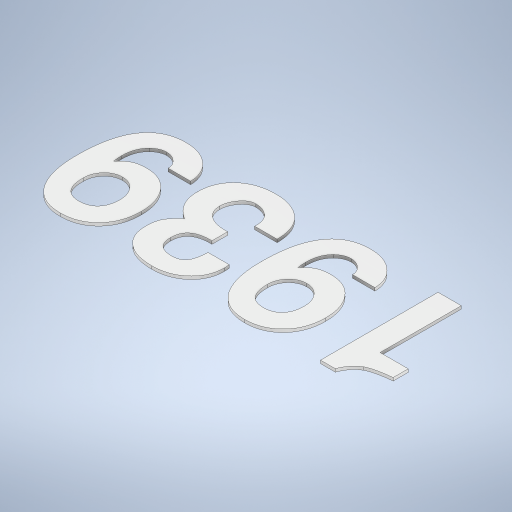
# Autodesk Inventor part: Numbers
Saved by Autodesk Inventor 2023 (Build 270158000, 158)
## iProperties
Created: 2023-11-22
Part Number: Numbers
Material: Generic
Document SubType Name: Modeling
Designer: adamarnold
Density: 1 g/cm^3
Appearance: Default
Author: adamarnold
Autodesk Inventor part; units mm, degrees
ref_plane "YZ Plane" through (0, 0, 0) normal (1, 0, 0) x (0, 1, 0)
ref_plane "XZ Plane" through (0, 0, 0) normal (0, 1, 0) x (-1, 0, 0)
ref_plane "XY Plane" through (0, 0, 0) normal (0, 0, 1) x (1, 0, 0)
sketch "Sketch1" plane through (0, 0, 0) normal (0, 1, 0) x (-1, 0, 0)
  line L0 (0, 0.0214) -> (189.558, 0.0214) construction
  line L1 (189.558, 0.0214) -> (189.558, -78.5059) construction
  line L2 (189.558, -78.5059) -> (0, -78.5059) construction
  line L3 (0, -78.5059) -> (0, 0.0214) construction
  line L4 (26.3876, -50.5021) -> (16.6305, -50.5021)
  line L5 (16.6305, -50.5021) -> (16.6305, -16.3721)
  line L6 (16.6305, -16.3721) -> (4.7798, -16.3721)
  line L7 (4.7798, -16.3721) -> (4.7798, -10.0122)
  spline S0 degree 2 poles (4.7798, -10.0122) (11.8112, -9.3012) (14.8134, -7.7606) knots 0 0 0 1 1 1
  spline S1 degree 2 poles (14.8134, -7.7606) (18.2896, -5.904) (20.1857, -1.0847) knots 0 0 0 1 1 1
  line L8 (20.1857, -1.0847) -> (26.3876, -1.0847)
  line L9 (26.3876, -1.0847) -> (26.3876, -50.5021)
  spline S2 degree 2 poles (74.7384, -24.4306) (74.7384, -52.0427) (56.2513, -52.0427) knots 0 0 0 1 1 1
  spline S3 degree 2 poles (56.2513, -52.0427) (49.9309, -52.0427) (41.4774, -44.5767) (41.3589, -38.9279) knots 0 0 0 1 2 2 2
  line L10 (41.3589, -38.9279) -> (50.8395, -38.9279)
  spline S4 degree 2 poles (50.8395, -38.9279) (50.6815, -41.0215) (54.4737, -44.4977) (56.9624, -44.4977) knots 0 0 0 1 2 2 2
  spline S5 degree 2 poles (56.9624, -44.4977) (59.688, -44.4977) (62.0187, -42.2856) knots 0 0 0 1 1 1
  spline S6 degree 2 poles (62.0187, -42.2856) (65.1393, -39.3624) (65.1393, -33.7136) knots 0 0 0 1 1 1
  spline S7 degree 2 poles (65.1393, -33.7136) (65.1393, -31.9755) (64.8628, -30.0794) knots 0 0 0 1 1 1
  spline S8 degree 2 poles (64.8628, -30.0794) (62.5717, -32.5285) (60.8731, -33.3581) knots 0 0 0 1 1 1
  spline S9 degree 2 poles (60.8731, -33.3581) (58.7795, -34.4246) (55.3823, -34.4246) knots 0 0 0 1 1 1
  spline S10 degree 2 poles (55.3823, -34.4246) (48.6274, -34.4246) (44.6376, -29.5264) knots 0 0 0 1 1 1
  spline S11 degree 2 poles (44.6376, -29.5264) (40.7269, -24.8651) (40.7269, -17.5572) knots 0 0 0 1 1 1
  spline S12 degree 2 poles (40.7269, -17.5572) (40.7269, -9.6567) (49.9309, 0.0214) (57.1599, 0.0214) knots 0 0 0 1 2 2 2
  spline S13 degree 2 poles (57.1599, 0.0214) (66.4429, 0.0214) (70.9857, -7.5236) knots 0 0 0 1 1 1
  spline S14 degree 2 poles (70.9857, -7.5236) (74.7384, -13.8439) (74.7384, -24.4306) knots 0 0 0 1 1 1
  spline S15 degree 2 poles (65.1393, -17.5572) (65.1393, -8.1951) (57.5944, -8.1951) knots 0 0 0 1 1 1
  spline S16 degree 2 poles (57.5944, -8.1951) (53.7232, -8.1951) (49.4569, -13.0144) (49.4569, -17.2806) knots 0 0 0 1 2 2 2
  spline S17 degree 2 poles (49.4569, -17.2806) (49.4569, -21.1124) (53.8812, -26.1292) (57.1599, -26.1292) knots 0 0 0 1 2 2 2
  spline S18 degree 2 poles (57.1599, -26.1292) (60.5176, -26.1292) (65.1393, -21.1124) (65.1393, -17.5572) knots 0 0 0 1 2 2 2
  spline S19 degree 2 poles (113.5692, -36.3603) (113.5692, -43.5892) (104.0886, -52.1612) (96.1487, -52.1612) knots 0 0 0 1 2 2 2
  spline S20 degree 2 poles (96.1487, -52.1612) (89.5123, -52.1612) (85.0485, -48.685) knots 0 0 0 1 1 1
  spline S21 degree 2 poles (85.0485, -48.685) (79.5577, -44.3792) (79.5577, -36.0047) knots 0 0 0 1 1 1
  line L11 (79.5577, -36.0047) -> (89.0383, -36.0047)
  spline S22 degree 2 poles (89.0383, -36.0047) (88.6827, -40.3105) (91.5664, -42.6016) knots 0 0 0 1 1 1
  spline S23 degree 2 poles (91.5664, -42.6016) (93.7785, -44.4187) (96.9782, -44.4187) knots 0 0 0 1 1 1
  spline S24 degree 2 poles (96.9782, -44.4187) (99.5854, -44.4187) (103.6936, -39.0464) (103.6936, -36.0442) knots 0 0 0 1 2 2 2
  spline S25 degree 2 poles (103.6936, -36.0442) (103.6936, -32.252) (97.7683, -28.1043) (92.6725, -28.3413) knots 0 0 0 1 2 2 2
  line L12 (92.6725, -28.3413) -> (92.6725, -21.7049)
  spline S26 degree 2 poles (92.6725, -21.7049) (102.5481, -21.9814) (102.5481, -14.1995) knots 0 0 0 1 1 1
  spline S27 degree 2 poles (102.5481, -14.1995) (102.5481, -7.7211) (95.7142, -7.7211) knots 0 0 0 1 1 1
  spline S28 degree 2 poles (95.7142, -7.7211) (92.6725, -7.7211) (91.2504, -9.2617) knots 0 0 0 1 1 1
  spline S29 degree 2 poles (91.2504, -9.2617) (89.4333, -11.2763) (89.2358, -16.6486) knots 0 0 0 1 1 1
  line L13 (89.2358, -16.6486) -> (80.3082, -16.6486)
  spline S30 degree 2 poles (80.3082, -16.6486) (80.1897, -15.5425) (80.1897, -14.476) knots 0 0 0 1 1 1
  spline S31 degree 2 poles (80.1897, -14.476) (80.1897, -8.0766) (89.3148, 0.0214) (96.2672, 0.0214) knots 0 0 0 1 2 2 2
  spline S32 degree 2 poles (96.2672, 0.0214) (103.2591, 0.0214) (107.4068, -3.2573) knots 0 0 0 1 1 1
  spline S33 degree 2 poles (107.4068, -3.2573) (111.9496, -6.7335) (111.9496, -13.2119) knots 0 0 0 1 1 1
  spline S34 degree 2 poles (111.9496, -13.2119) (111.9496, -16.9646) (110.6855, -19.2953) knots 0 0 0 1 1 1
  spline S35 degree 2 poles (110.6855, -19.2953) (109.6585, -21.0729) (106.5378, -23.996) knots 0 0 0 1 1 1
  spline S36 degree 2 poles (106.5378, -23.996) (113.5692, -28.5388) (113.5692, -36.3603) knots 0 0 0 1 1 1
  spline S37 degree 2 poles (152.242, -24.4306) (152.242, -52.0427) (133.7549, -52.0427) knots 0 0 0 1 1 1
  spline S38 degree 2 poles (133.7549, -52.0427) (127.4345, -52.0427) (118.981, -44.5767) (118.8625, -38.9279) knots 0 0 0 1 2 2 2
  line L14 (118.8625, -38.9279) -> (128.3431, -38.9279)
  spline S39 degree 2 poles (128.3431, -38.9279) (128.1851, -41.0215) (131.9773, -44.4977) (134.4659, -44.4977) knots 0 0 0 1 2 2 2
  spline S40 degree 2 poles (134.4659, -44.4977) (137.1916, -44.4977) (139.5222, -42.2856) knots 0 0 0 1 1 1
  spline S41 degree 2 poles (139.5222, -42.2856) (142.6429, -39.3624) (142.6429, -33.7136) knots 0 0 0 1 1 1
  spline S42 degree 2 poles (142.6429, -33.7136) (142.6429, -31.9755) (142.3664, -30.0794) knots 0 0 0 1 1 1
  spline S43 degree 2 poles (142.3664, -30.0794) (140.0753, -32.5285) (138.3767, -33.3581) knots 0 0 0 1 1 1
  spline S44 degree 2 poles (138.3767, -33.3581) (136.283, -34.4246) (132.8858, -34.4246) knots 0 0 0 1 1 1
  spline S45 degree 2 poles (132.8858, -34.4246) (126.1309, -34.4246) (122.1412, -29.5264) knots 0 0 0 1 1 1
  spline S46 degree 2 poles (122.1412, -29.5264) (118.2305, -24.8651) (118.2305, -17.5572) knots 0 0 0 1 1 1
  spline S47 degree 2 poles (118.2305, -17.5572) (118.2305, -9.6567) (127.4345, 0.0214) (134.6635, 0.0214) knots 0 0 0 1 2 2 2
  spline S48 degree 2 poles (134.6635, 0.0214) (143.9465, 0.0214) (148.4893, -7.5236) knots 0 0 0 1 1 1
  spline S49 degree 2 poles (148.4893, -7.5236) (152.242, -13.8439) (152.242, -24.4306) knots 0 0 0 1 1 1
  spline S50 degree 2 poles (142.6429, -17.5572) (142.6429, -8.1951) (135.098, -8.1951) knots 0 0 0 1 1 1
  spline S51 degree 2 poles (135.098, -8.1951) (131.2267, -8.1951) (126.9605, -13.0144) (126.9605, -17.2806) knots 0 0 0 1 2 2 2
  spline S52 degree 2 poles (126.9605, -17.2806) (126.9605, -21.1124) (131.3848, -26.1292) (134.6635, -26.1292) knots 0 0 0 1 2 2 2
  spline S53 degree 2 poles (134.6635, -26.1292) (138.0211, -26.1292) (142.6429, -21.1124) (142.6429, -17.5572) knots 0 0 0 1 2 2 2
  point P0 (0, 0)
  constraints: 2 other
extrude "Extrusion1" add sketch "Sketch1" along normal blind 1.27
body "Solid1"
